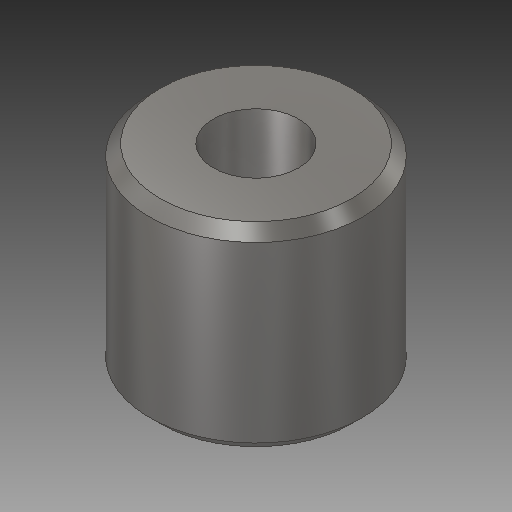
# Autodesk Inventor part: ARU-304S
Saved by Autodesk Inventor 2018 (Build 220112000, 112)
## iProperties
Created: 2016-08-23
Part Number: ARU-304S
Material: ステンレス鋼 440C
Document SubType Name: Modeling
Designer: hiro
Density: 7.75 g/cm^3
Appearance: 半つや出し
Mass: 0.999653 g
Surface Area: 1.85783 cm^2
Volume: 0.128988 cm^3
Author: hiro
Autodesk Inventor part; units mm, degrees
ref_plane "YZ Plane" through (0, 0, 0) normal (1, 0, 0) x (0, 1, 0)
ref_plane "XZ Plane" through (0, 0, 0) normal (0, 1, 0) x (-1, 0, 0)
ref_plane "XY Plane" through (0, 0, 0) normal (0, 0, 1) x (1, 0, 0)
sketch "スケッチ1" plane through (0, 0, 0) normal (0, 0, 1) x (1, 0, 0)
  line L0 (1.2, -2.75) -> (1.2, 2.75)
  line L1 (1.2, 2.75) -> (2.7, 2.75)
  line L2 (2.7, 2.75) -> (3, 2.45)
  line L3 (3, 2.45) -> (3, -2.45)
  line L4 (0, 6.6667) -> (0, -6.6667) construction
  line L5 (3, -2.45) -> (2.7, -2.75)
  line L6 (2.7, -2.75) -> (1.2, -2.75)
  point P0 (0, 0)
  point P1 (0, 0)
  point P2 (1.2, 0)
  point P3 (3, 0)
  dimension "d0" = 6
  dimension "d1" = 2.4
  dimension "d3" = 5.5
  dimension "d4" = 0.3
  dimension "d5" = 0.3
  constraints: 14 end point, 3 midpoint, 2 horizontal alignment, 2 perpendicular, 1 coincident, 1 horizontal, 1 parallel, 1 vertical
  measures "d0" diameter of L3 L4
  measures "d1" diameter of L0 L4
  measures "d3" distance between parallel lines of L6 L1
  measures "d4" horizontal distance of L2.end L1.end
  measures "d5" horizontal distance of L1.end L2.end
revolve "回転1" add sketch "スケッチ1" angle 360 about axis through (0, 6.6667, 0) along (0, -1, 0)
equation "\"d5\" = d4"
